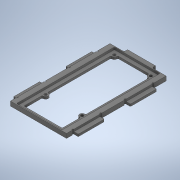
# Autodesk Inventor part: Cockpit_horizontal_frame_01
Saved by Autodesk Inventor 2020.4 (Build 244396000, 396)
## iProperties
Created: 2021-04-14
Part Number: Cockpit_horizontal_frame_01
Material: アセタール樹脂、黒
Document SubType Name: Modeling
Designer: Masato Kubotera
Density: 1.425 g/cm^3
Appearance: 滑らか - 黒
Mass: 18.0359 g
Surface Area: 107.499 cm^2
Volume: 12.6568 cm^3
Description: POM T5
Author: Masato Kubotera
Title: Cockpit_horizontal_frame_01
Autodesk Inventor part; units mm, degrees
ref_plane "YZ Plane" through (0, 0, 0) normal (1, 0, 0) x (0, 1, 0)
ref_plane "XZ Plane" through (0, 0, 0) normal (0, 1, 0) x (-1, 0, 0)
ref_plane "XY Plane" through (0, 0, 0) normal (0, 0, 1) x (1, 0, 0)
sketch "スケッチ1" plane through (0, 0, 0) normal (0, 0, 1) x (1, 0, 0)
  line L0 (-32.25, 65) -> (-16, 65) construction
  line L1 (32.25, 65) -> (32.25, 61) construction
  line L2 (-32.25, -65) -> (-32.25, -47.1)
  line L3 (-32.25, 65) -> (32.25, -65) construction
  line L4 (32.25, 65) -> (-32.25, -65) construction
  line L5 (-32.25, 45) -> (-37.25, 45)
  line L6 (-37.25, 15) -> (-32.25, 15)
  line L7 (-37.25, 15) -> (-37.25, 45)
  line L8 (-32.25, -15) -> (-37.25, -15)
  line L9 (-37.25, -15) -> (-37.25, -45)
  line L10 (-37.25, -45) -> (-32.25, -45)
  arc A0 (-32.25, 45) -> (-32.25, 47.1) centre (-32.25, 46.05) ccw
  arc A1 (-32.25, 12.9) -> (-32.25, 15) centre (-32.25, 13.95) ccw
  arc A2 (-32.25, -15) -> (-32.25, -12.9) centre (-32.25, -13.95) ccw
  arc A3 (-32.25, -47.1) -> (-32.25, -45) centre (-32.25, -46.05) ccw
  line L11 (-32.25, 47.1) -> (-32.25, 61)
  line L12 (-32.25, 12.9) -> (-32.25, 15) construction
  line L13 (-32.25, -12.9) -> (-32.25, 12.9)
  line L14 (-32.25, -47.1) -> (-32.25, -45) construction
  line L15 (0, 64.25) -> (0, -85.6509) construction
  arc A4 (32.25, -45) -> (32.25, -47.1) centre (32.25, -46.05) ccw
  line L16 (37.25, -45) -> (32.25, -45)
  line L17 (37.25, -15) -> (37.25, -45)
  line L18 (32.25, -15) -> (37.25, -15)
  arc A5 (32.25, -12.9) -> (32.25, -15) centre (32.25, -13.95) ccw
  arc A6 (32.25, 15) -> (32.25, 12.9) centre (32.25, 13.95) ccw
  line L19 (37.25, 15) -> (37.25, 45)
  line L20 (37.25, 15) -> (32.25, 15)
  line L21 (32.25, 45) -> (37.25, 45)
  arc A7 (32.25, 47.1) -> (32.25, 45) centre (32.25, 46.05) ccw
  line L22 (32.25, 47.1) -> (32.25, 45) construction
  line L23 (32.25, 12.9) -> (32.25, -12.9)
  line L24 (32.25, -47.1) -> (32.25, -65)
  line L25 (32.25, -12.9) -> (32.25, -15) construction
  line L26 (-32.25, -15) -> (-32.25, -12.9) construction
  line L27 (-32.25, -45) -> (-32.25, -15)
  line L28 (32.25, -15) -> (32.25, -45)
  line L29 (32.25, -45) -> (32.25, -47.1) construction
  line L30 (-32.25, -65) -> (32.25, -65) construction
  line L31 (-32.25, 45) -> (-32.25, 47.1) construction
  line L32 (-32.25, 15) -> (-32.25, 45)
  line L33 (32.25, 15) -> (32.25, 12.9) construction
  line L34 (32.25, 45) -> (32.25, 15)
  line L35 (-25, -51.25) -> (25, -51.25) construction
  line L36 (25, -51.25) -> (25, 58.75) construction
  line L37 (25, 58.75) -> (-25, 58.75) construction
  line L38 (-25, 58.75) -> (-25, -51.25) construction
  line L39 (-25, -51.25) -> (25, 58.75) construction
  line L40 (25, -51.25) -> (-25, 58.75) construction
  circle A8 centre (-21, 54.75) radius 1.55
  circle A9 centre (-21, -24.25) radius 1.55
  circle A10 centre (21, 54.75) radius 1.55
  circle A11 centre (21, -24.25) radius 1.55
  line L41 (-22, -48.25) -> (22, -48.25)
  line L42 (22, -48.25) -> (22, -27.0784)
  line L43 (22, 55.75) -> (18.1716, 55.75) construction
  line L44 (-22, 55.75) -> (-22, 51.9216) construction
  line L45 (-22, -48.25) -> (22, 55.75) construction
  line L46 (22, -48.25) -> (-22, 55.75) construction
  arc A12 (-22, -27.0784) -> (-22, -21.4216) centre (-21, -24.25) ccw
  arc A13 (-22, 51.9216) -> (-18.1716, 55.75) centre (-21, 54.75) ccw
  arc A14 (22, -21.4216) -> (22, -27.0784) centre (21, -24.25) ccw
  arc A15 (18.1716, 55.75) -> (22, 51.9216) centre (21, 54.75) ccw
  line L47 (-22, -21.4216) -> (-22, -27.0784) construction
  line L48 (-22, -27.0784) -> (-22, -48.25)
  line L49 (-18.1716, 55.75) -> (-22, 55.75) construction
  line L50 (-22, 51.9216) -> (-22, -21.4216)
  line L51 (18.1716, 55.75) -> (-18.1716, 55.75)
  line L52 (22, 51.9216) -> (22, 55.75) construction
  line L53 (22, -27.0784) -> (22, -21.4216) construction
  line L54 (22, -21.4216) -> (22, 51.9216)
  line L55 (26.25, -52.5) -> (-26.25, -52.5)
  line L56 (-26.25, -52.5) -> (-26.25, 60)
  line L57 (-26.25, 60) -> (26.25, 60)
  line L58 (26.25, 60) -> (26.25, -52.5)
  line L59 (26.25, -52.5) -> (-26.25, 60) construction
  line L60 (-26.25, -52.5) -> (26.25, 60) construction
  line L61 (-32.25, 61) -> (-16, 61)
  line L62 (-16, 61) -> (-16, 65)
  line L63 (32.25, 61) -> (16, 61)
  line L64 (16, 61) -> (16, 65)
  line L65 (16, 65) -> (32.25, 65) construction
  line L66 (-16, 65) -> (16, 65)
  line L67 (-32.25, 61) -> (-32.25, 65) construction
  line L68 (32.25, 61) -> (32.25, 47.1)
  line L69 (-32.25, -65) -> (-32.25, -70)
  line L70 (-32.25, -70) -> (32.25, -70)
  line L71 (32.25, -70) -> (32.25, -65)
  line L72 (-32.25, -53.5) -> (32.25, -53.5)
  point P0 (0, 0)
  point P1 (0, 0)
  point P2 (0, 0)
  point P3 (0, 0)
  point P4 (0, 0)
  point P5 (28, 15)
  point P6 (28, 45)
  point P7 (28, 15)
  point P8 (28, 45)
  point P9 (0, 3.75)
  point P10 (28, 61)
  dimension "d0" = 64.5
  dimension "d2" = 20
  dimension "d3" = 30
  dimension "d4" = 30
  dimension "d5" = 30
  dimension "d6" = 1.05
  dimension "d7" = 1.05
  dimension "d8" = 1.05
  dimension "d9" = 1.05
  dimension "d10" = 5
  dimension "d48" = 110
  dimension "d49" = 3.1
  dimension "d50" = 79
  dimension "d51" = 3.1
  dimension "d52" = 42
  dimension "d53" = 42
  dimension "d54" = 4
  dimension "d55" = 3
  dimension "d56" = 3
  dimension "d57" = 3
  dimension "d58" = 3
  dimension "d59" = 50
  dimension "d60" = 1.25
  dimension "d61" = 1.25
  dimension "d73" = 130
  dimension "d74" = 32
  dimension "d75" = 4
  dimension "d77" = 1
  dimension "d78" = 5
  dimension "d80" = 1
  constraints: 144 end point, 113 parallel, 69 perpendicular, 27 symmetric about line, 24 point on circle, 16 centre point, 14 midpoint, 12 horizontal, 11 vertical, 5 point on line, 4 coincident, 1 collinear, 23 other
  measures "d0" distance of L3.start L4.start
  measures "d2" distance between parallel lines of L5 L0
  measures "d3" distance of L6.start L5.end
  measures "d4" distance between parallel lines of L8 L6
  measures "d5" distance of L8.end L9.end
  measures "d6" radius of A0
  measures "d7" radius of A1
  measures "d8" radius of A2
  measures "d9" radius of A3
  measures "d10" distance between parallel lines of L7 L11
  measures "d48" distance of L35.end L36.end
  measures "d49" diameter of A8
  measures "d50" distance of A9.centre A8.centre
  measures "d51" diameter of A9
  measures "d52" distance of A10.centre A8.centre
  measures "d53" distance of A11.centre A9.centre
  measures "d54" distance from line of L37 A8.centre
  measures "d55" distance between parallel lines of L38 L44
  measures "d56" distance between parallel lines of L35 L41
  measures "d57" radius of A13
  measures "d58" radius of A12
  measures "d59" distance between parallel lines of L38 L36
  measures "d60" distance between parallel lines of L35 L55
  measures "d61" distance between parallel lines of L38 L56
  measures "d73" distance of L4.start L3.end
  measures "d74" distance of L0.end L64.end
  measures "d75" distance of L61.end L0.end
  measures "d77" distance from line of L57 L11.end
  measures "d78" distance of L4.end L69.end
  measures "d80" vertical distance of L72.start L55.end
extrude "押し出し1" add sketch "スケッチ1" along normal blind 2.5 contours L2 A3 L27 A2 L13 A1 L32 A0 L11 L61 L62 L66 L64 L63 L68 A7 L34 A6 L23 A5 L28 A4 L24 L72 | L10 L9 L8 L27 | L28 L18 L17 L16 | L6 L7 L5 L32 | L34 L21 L19 L20 | L55 L56 L57 L58
extrude "押し出し2" add sketch "スケッチ1" along normal blind 5 contours L2 A3 L27 A2 L13 A1 L32 A0 L11 L61 L62 L66 L64 L63 L68 A7 L34 A6 L23 A5 L28 A4 L24 L72
fillet "フィレット1" radius 1 14 edges at (-22, -48.25, 1.25) (-18.1716, 55.75, 1.25) (-22, 51.9216, 1.25) (-22, -27.0784, 1.25) (-22, -21.4216, 1.25) (18.1716, 55.75, 1.25) (22, 51.9216, 1.25) (22, -27.0784, 1.25) (22, -21.4216, 1.25) (22, -48.25, 1.25) (26.25, -52.5, 3.75) (-26.25, -52.5, 3.75) (26.25, 60, 3.75) (-26.25, 60, 3.75)
fillet "フィレット2" radius 2 2 edges at (16, 61, 2.5) (-16, 61, 2.5)
chamfer "面取り1" distance 0.5 angle 45 8 edges at (-37.25, -45, 1.25) (37.25, -45, 1.25) (37.25, -15, 1.25) (37.25, 15, 1.25) (37.25, 45, 1.25) (-37.25, 45, 1.25) (-37.25, 15, 1.25) (-37.25, -15, 1.25)
equation "\"d2\" = -0.5 * d4 + 0.5 * d1 - d3"
equation "\"d5\" = d3"
equation "\"d7\" = d6"
equation "\"d8\" = d7"
equation "\"d9\" = d8"
equation "\"d51\" = d49"
equation "\"d53\" = d52"
equation "\"d56\" = d55"
equation "\"d58\" = d57"
equation "\"d61\" = d60"
equation "\"d1\" = 130"
